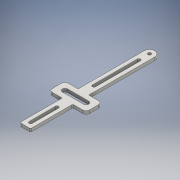
# Autodesk Inventor part: Slider_1
Saved by Autodesk Inventor 2016 (Build 200138000, 138)
## iProperties
Created: 2015-12-09
Part Number: Slider_1
Material: Generic
Document SubType Name: Modeling
Designer: lk8187
Density: 1 g/cm^3
Appearance: Smooth - White
Author: lk8187
Autodesk Inventor part; units mm, degrees
ref_plane "YZ Plane" through (0, 0, 0) normal (1, 0, 0) x (0, 1, 0)
ref_plane "XZ Plane" through (0, 0, 0) normal (0, 1, 0) x (-1, 0, 0)
ref_plane "XY Plane" through (0, 0, 0) normal (0, 0, 1) x (1, 0, 0)
sketch "Sketch1" plane through (0, 0, 0) normal (0, 0, 1) x (1, 0, 0)
  line L0 (-10, 0) -> (10, 0) construction
  line L1 (-10, -2.5) -> (10, -2.5)
  line L2 (10, 2.5) -> (-10, 2.5)
  arc A0 (-10, 2.5) -> (-10, -2.5) centre (-10, 0) ccw
  arc A1 (10, -2.5) -> (10, 2.5) centre (10, 0) ccw
  line L3 (17.5, 4.5) -> (17.5, -4.5)
  line L4 (-17.5, -4.5) -> (-17.5, 4.5)
  line L5 (-5, 70) -> (5, 70) construction
  line L6 (5, 70) -> (5, 8.5)
  line L7 (-5, 7.5) -> (-5, 7.5)
  line L8 (-5, 8.5) -> (-5, 70)
  line L9 (5, -7.5) -> (5, -7.5)
  line L10 (5, -8.5) -> (5, -42.5)
  line L11 (5, -42.5) -> (-5, -42.5) construction
  line L12 (-5, -42.5) -> (-5, -8.5)
  line L13 (14.5, -7.5) -> (6, -7.5)
  line L14 (-6, -7.5) -> (-14.5, -7.5)
  line L15 (-14.5, 7.5) -> (-6, 7.5)
  line L16 (6, 7.5) -> (14.5, 7.5)
  arc A2 (5, 70) -> (-5, 70) centre (0, 70) ccw
  circle A3 centre (0, 70) radius 1.5
  line L17 (0, 60) -> (0, 17.5) construction
  line L18 (-1.5, 60) -> (-1.5, 17.5)
  line L19 (1.5, 17.5) -> (1.5, 60)
  arc A4 (1.5, 60) -> (-1.5, 60) centre (0, 60) ccw
  arc A5 (-1.5, 17.5) -> (1.5, 17.5) centre (0, 17.5) ccw
  arc A6 (-5, -42.5) -> (5, -42.5) centre (0, -42.5) ccw construction
  line L20 (0, -42.5) -> (0, -17.5) construction
  line L21 (-1.5, -42.5) -> (-1.5, -17.5)
  line L22 (1.5, -17.5) -> (1.5, -42.5)
  arc A7 (-1.5, -42.5) -> (1.5, -42.5) centre (0, -42.5) ccw
  arc A8 (1.5, -17.5) -> (-1.5, -17.5) centre (0, -17.5) ccw
  arc A9 (17.5, 4.5) -> (14.5, 7.5) centre (14.5, 4.5) ccw
  arc A10 (14.5, -7.5) -> (17.5, -4.5) centre (14.5, -4.5) ccw
  arc A11 (-17.5, -4.5) -> (-14.5, -7.5) centre (-14.5, -4.5) ccw
  arc A12 (-14.5, 7.5) -> (-17.5, 4.5) centre (-14.5, 4.5) ccw
  arc A13 (-5, -8.5) -> (-6, -7.5) centre (-6, -8.5) ccw
  arc A14 (6, -7.5) -> (5, -8.5) centre (6, -8.5) ccw
  arc A15 (5, 8.5) -> (6, 7.5) centre (6, 8.5) ccw
  arc A16 (-6, 7.5) -> (-5, 8.5) centre (-6, 8.5) ccw
  line L23 (5, -42.5) -> (5, -46.5)
  line L24 (4, -47.5) -> (-4, -47.5)
  line L25 (-5, -46.5) -> (-5, -42.5)
  arc A17 (4, -47.5) -> (5, -46.5) centre (4, -46.5) ccw
  arc A18 (-5, -46.5) -> (-4, -47.5) centre (-4, -46.5) ccw
  point P0 (0, 0)
  point P1 (0, 2.5)
  point P2 (-17.5, 0)
  point P3 (17.5, 0)
  point P4 (0, 38.75)
  point P5 (0, -30)
  dimension "d0" = 10
  dimension "d1" = 35
  dimension "d2" = 15
  dimension "d3" = 5
  dimension "d4" = 20
  dimension "d5" = 3
  dimension "d6" = 10
  dimension "d7" = 10
  dimension "d8" = 70
  dimension "d9" = 3
  dimension "d10" = 35
  dimension "d11" = 3
  dimension "d12" = 10
  dimension "d13" = 3
  dimension "d14" = 1
  dimension "d17" = 1
  constraints: 58 end point, 37 tangent, 36 point on circle, 19 centre point, 13 parallel, 7 equal radius, 7 midpoint, 7 point on line, 6 perpendicular, 5 horizontal, 4 collinear, 2 horizontal alignment, 2 vertical, 2 vertical alignment, 1 coincident
  measures "d0" distance between parallel lines of L6 L8
  measures "d1" distance between parallel lines of L3 L4
  measures "d2" distance between parallel lines of L13 L16
  measures "d3" distance between parallel lines of L1 L2
  measures "d4" distance of L0.start L0.end
  measures "d5" distance between parallel lines of L18 L19
  measures "d6" distance of point (0, 70) L17.start
  measures "d7" distance from line of L16 L17.end
  measures "d8" distance from line of point (0, 70) L0
  measures "d9" diameter of A3
  measures "d10" distance between parallel lines of L11 L13
  measures "d11" distance between parallel lines of L21 L22
  measures "d12" distance from line of L20.end L13
  measures "d13" radius of A9
  measures "d14" radius of A13
  measures "d17" radius of A17
extrude "Extrusion1" add sketch "Sketch1" against normal blind 3
body "Solid1"
